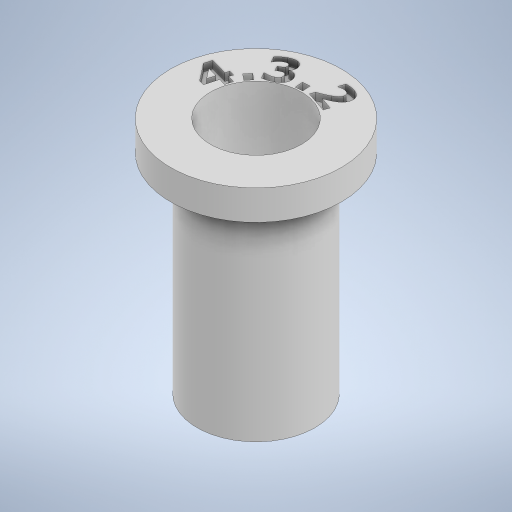
# Autodesk Inventor part: PancakeBearingAdapter
Saved by Autodesk Inventor 2024.3 (Build 283343000, 343)
## iProperties
Created: 2024-12-03
Part Number: PancakeBearingAdapter
Material: Generisch
Document SubType Name: Modeling
Designer: Maximilian Hock
Density: 1 g/cm^3
Appearance: Vorgabe
Author: Maximilian Hock
## iProperties of the stored document MemberDocs/xG1cw44kiPcn4fagy3cfzayvmYe
Created: 2024-12-03
Part Number: PancakeBearingAdapter
Material: Generisch
Document SubType Name: Modeling
Designer: Maximilian Hock
Density: 1 g/cm^3
Appearance: Vorgabe
Author: Maximilian Hock
Autodesk Inventor part; units mm, degrees
ref_plane "YZ Plane" through (0, 0, 0) normal (1, 0, 0) x (0, 1, 0)
ref_plane "XZ Plane" through (0, 0, 0) normal (0, 1, 0) x (-1, 0, 0)
ref_plane "XY Plane" through (0, 0, 0) normal (0, 0, 1) x (1, 0, 0)
sketch "Skizze1" plane through (0, 0, 0) normal (0, 0, 1) x (1, 0, 0)
  circle A0 centre (0, 0) radius 7.5 construction
  circle A1 centre (0, 0) radius 3.95
  circle A2 centre (0, 0) radius 3.05
  line L0 (0, 3.95) -> (0, 7.5) construction
  circle A3 centre (0, 0) radius 5.725
  point P0 (0, 5.725)
  dimension "d1" = 7.9
  dimension "d2" = 15
  dimension "d0" = 6.1
  constraints: 4 coincident, 3 vertical alignment, 2 end point, 2 vertical, 1 centre point, 1 midpoint, 6 other
  measures "d0" diameter of A2
extrude "Extrusion1" add sketch "Skizze1" against normal blind 14 contours A1
extrude "Extrusion2" add sketch "Skizze1" along normal blind 2 contours A1 | A3
sketch "Skizze3" plane through (0, 0, 2) normal (0, 0, 1) x (1, 0, 0)
  circle A0 centre (0, 0) radius 5.725 projected
  circle A1 centre (0, 0) radius 3.05 projected
  line L0 (-3.2646, 1.7599) -> (-3.3371, 1.4992)
  line L1 (-3.3371, 1.4992) -> (-2.8827, 1.3728)
  line L2 (-2.8827, 1.3728) -> (-3.0126, 0.9059)
  line L3 (-3.0126, 0.9059) -> (-3.467, 1.0323)
  line L4 (-3.467, 1.0323) -> (-3.7032, 0.1828)
  line L5 (-3.7032, 0.1828) -> (-4.0623, 0.2827)
  line L6 (-4.0623, 0.2827) -> (-4.9485, 1.4275)
  line L7 (-4.9485, 1.4275) -> (-4.8143, 1.91)
  line L8 (-4.8143, 1.91) -> (-3.6838, 1.5956)
  line L9 (-3.6838, 1.5956) -> (-3.6112, 1.8563)
  line L10 (-3.6112, 1.8563) -> (-3.2646, 1.7599)
  line L11 (-3.8136, 1.1287) -> (-4.4694, 1.3111)
  line L12 (-4.4694, 1.3111) -> (-3.9495, 0.6399)
  line L13 (-3.9495, 0.6399) -> (-3.8136, 1.1287)
  line L14 (-2.3049, 2.1601) -> (-2.6027, 1.7902)
  line L15 (-2.6027, 1.7902) -> (-3.0142, 2.1217)
  line L16 (-3.0142, 2.1217) -> (-2.7164, 2.4915)
  line L17 (-2.7164, 2.4915) -> (-2.3049, 2.1601)
  spline S0 degree 2 poles (-1.0947, 3.6698) (-1.0258, 3.5394) (-1.009, 3.2751) (-1.0628, 3.1514) knots 0 0 0 1 2 2 2
  spline S1 degree 2 poles (-1.0628, 3.1514) (-1.1165, 3.0277) (-1.3278, 2.8134) (-1.5098, 2.7173) knots 0 0 0 1 2 2 2
  spline S2 degree 2 poles (-1.5098, 2.7173) (-1.7162, 2.6083) (-2.0477, 2.5211) (-2.1636, 2.5149) knots 0 0 0 1 2 2 2
  line L18 (-2.1636, 2.5149) -> (-2.3665, 2.8989)
  line L19 (-2.3665, 2.8989) -> (-2.3235, 2.9216)
  spline S3 degree 2 poles (-2.3235, 2.9216) (-2.1935, 2.9115) (-1.8828, 2.9583) (-1.7739, 3.0159) knots 0 0 0 1 2 2 2
  spline S4 degree 2 poles (-1.7739, 3.0159) (-1.7094, 3.0499) (-1.571, 3.1524) (-1.5391, 3.2169) knots 0 0 0 1 2 2 2
  spline S5 degree 2 poles (-1.5391, 3.2169) (-1.5149, 3.2682) (-1.5123, 3.3813) (-1.554, 3.4601) knots 0 0 0 1 2 2 2
  spline S6 degree 2 poles (-1.554, 3.4601) (-1.5956, 3.539) (-1.7091, 3.5872) (-1.777, 3.577) knots 0 0 0 1 2 2 2
  spline S7 degree 2 poles (-1.777, 3.577) (-1.8449, 3.5667) (-2.0063, 3.487) (-2.0679, 3.4544) knots 0 0 0 1 2 2 2
  line L20 (-2.0679, 3.4544) -> (-2.1438, 3.4143)
  line L21 (-2.1438, 3.4143) -> (-2.3081, 3.7253)
  line L22 (-2.3081, 3.7253) -> (-2.2379, 3.7624)
  spline S8 degree 2 poles (-2.2379, 3.7624) (-2.1576, 3.8048) (-2.0291, 3.891) (-1.9931, 3.9375) knots 0 0 0 1 2 2 2
  spline S9 degree 2 poles (-1.9931, 3.9375) (-1.958, 3.9854) (-1.9473, 4.0937) (-1.9837, 4.1625) knots 0 0 0 1 2 2 2
  spline S10 degree 2 poles (-1.9837, 4.1625) (-2.0124, 4.2169) (-2.0982, 4.2578) (-2.1439, 4.2575) knots 0 0 0 1 2 2 2
  spline S11 degree 2 poles (-2.1439, 4.2575) (-2.1982, 4.2563) (-2.3204, 4.21) (-2.3605, 4.1888) knots 0 0 0 1 2 2 2
  spline S12 degree 2 poles (-2.3605, 4.1888) (-2.425, 4.1548) (-2.5453, 4.0528) (-2.5955, 3.9951) knots 0 0 0 1 2 2 2
  spline S13 degree 2 poles (-2.5955, 3.9951) (-2.6358, 3.9499) (-2.7129, 3.8322) (-2.7304, 3.8028) knots 0 0 0 1 2 2 2
  line L23 (-2.7304, 3.8028) -> (-2.7676, 3.7831)
  line L24 (-2.7676, 3.7831) -> (-2.9675, 4.1615)
  spline S14 degree 2 poles (-2.9675, 4.1615) (-2.8962, 4.2486) (-2.6253, 4.4852) (-2.4633, 4.5708) knots 0 0 0 1 2 2 2
  spline S15 degree 2 poles (-2.4633, 4.5708) (-2.3057, 4.6541) (-2.0448, 4.7223) (-1.9351, 4.7124) knots 0 0 0 1 2 2 2
  spline S16 degree 2 poles (-1.9351, 4.7124) (-1.8153, 4.7042) (-1.6341, 4.5799) (-1.5774, 4.4724) knots 0 0 0 1 2 2 2
  spline S17 degree 2 poles (-1.5774, 4.4724) (-1.4971, 4.3205) (-1.5523, 4.0018) (-1.6782, 3.8931) knots 0 0 0 1 2 2 2
  line L25 (-1.6782, 3.8931) -> (-1.6691, 3.8759)
  spline S18 degree 2 poles (-1.6691, 3.8759) (-1.6015, 3.9006) (-1.4569, 3.9183) (-1.3724, 3.897) knots 0 0 0 1 2 2 2
  spline S19 degree 2 poles (-1.3724, 3.897) (-1.2951, 3.8792) (-1.1477, 3.7701) (-1.0947, 3.6698) knots 0 0 0 1 2 2 2
  line L26 (-0.0136, 3.1588) -> (-0.487, 3.1212)
  line L27 (-0.487, 3.1212) -> (-0.5288, 3.6479)
  line L28 (-0.5288, 3.6479) -> (-0.0554, 3.6855)
  line L29 (-0.0554, 3.6855) -> (-0.0136, 3.1588)
  line L30 (1.7675, 2.7264) -> (0.3756, 3.1992)
  line L31 (0.3756, 3.1992) -> (0.4804, 3.5077)
  spline S20 degree 2 poles (0.4804, 3.5077) (0.7048, 3.5889) (1.0716, 3.7416) (1.2156, 3.8176) knots 0 0 0 1 2 2 2
  spline S21 degree 2 poles (1.2156, 3.8176) (1.4048, 3.916) (1.6047, 4.0963) (1.6443, 4.2129) knots 0 0 0 1 2 2 2
  spline S22 degree 2 poles (1.6443, 4.2129) (1.6891, 4.3449) (1.579, 4.5398) (1.4378, 4.5877) knots 0 0 0 1 2 2 2
  spline S23 degree 2 poles (1.4378, 4.5877) (1.3657, 4.6122) (1.2248, 4.6207) (1.1494, 4.6155) knots 0 0 0 1 2 2 2
  spline S24 degree 2 poles (1.1494, 4.6155) (1.0751, 4.6083) (0.9621, 4.5781) (0.9339, 4.5706) knots 0 0 0 1 2 2 2
  line L32 (0.9339, 4.5706) -> (0.8971, 4.5831)
  line L33 (0.8971, 4.5831) -> (1.0373, 4.9959)
  spline S25 degree 2 poles (1.0373, 4.9959) (1.1302, 5.0072) (1.4979, 4.9713) (1.656, 4.9176) knots 0 0 0 1 2 2 2
  spline S26 degree 2 poles (1.656, 4.9176) (1.9936, 4.8029) (2.2383, 4.3843) (2.146, 4.1126) knots 0 0 0 1 2 2 2
  spline S27 degree 2 poles (2.146, 4.1126) (2.0892, 3.9454) (1.8216, 3.6768) (1.5764, 3.5547) knots 0 0 0 1 2 2 2
  spline S28 degree 2 poles (1.5764, 3.5547) (1.4228, 3.4802) (1.1464, 3.3773) (1.0864, 3.3566) knots 0 0 0 1 2 2 2
  line L34 (1.0864, 3.3566) -> (1.889, 3.0839)
  line L35 (1.889, 3.0839) -> (1.7675, 2.7264)
  constraints: 1 other
emboss "Prägen2" sketch "Skizze3" operation cut depth 0.5 direction (0, 0, -1) contours L0 L1 L2 L3 L4 L5 L6 L7 L8 L9 L10 | L14 L15 L16 L17 | S0 S1 S2 L18 L19 S3 S4 S5 S6 S7 L20 L21 L22 S8 S9 S10 S11 S12 S13 L23 L24 S14 S15 S16 S17 L25 S18 S19 | L26 L27 L28 L29 | L30 L31 S20 S21 S22 S23 S24 L32 L33 S25 S26 S27 S28 L34 L35
equation "\"d1\" = BearingInnerDiameter - Clearance"
equation "\"d0\" = AxleDiameter + Clearance"
equation "\"d3\" = 2 * BearingHeight"
equation "\"BearingInnerDiameter\" = 8"
equation "\"Clearance\" = 0.1"
equation "\"AxleDiameter\" = 6"
equation "\"BearingHeight\" = 7"
